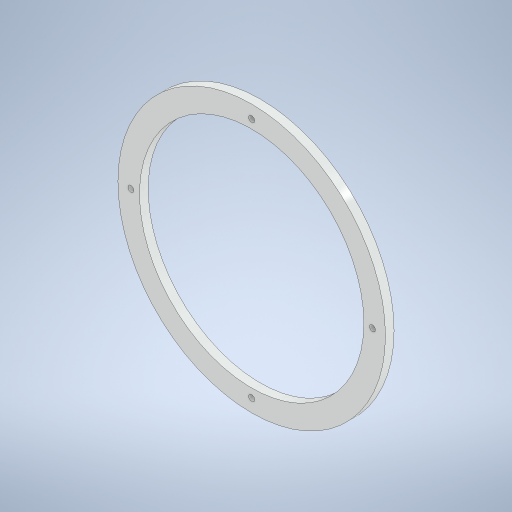
# Autodesk Inventor part: 아크릴 고정판
Saved by Autodesk Inventor 2023.1 (Build 271208000, 208)
## iProperties
Created: 2022-08-14
Part Number: 아크릴 고정판
Material: 일반
Document SubType Name: Modeling
Designer: fly01
Density: 1 g/cm^3
Appearance: 기본값
Author: fly01
Autodesk Inventor part; units mm, degrees
ref_plane "YZ Plane" through (0, 0, 0) normal (1, 0, 0) x (0, 1, 0)
ref_plane "XZ Plane" through (0, 0, 0) normal (0, 1, 0) x (-1, 0, 0)
ref_plane "XY Plane" through (0, 0, 0) normal (0, 0, 1) x (1, 0, 0)
sketch "스케치1" plane through (0, 0, 0) normal (0, 0, 1) x (1, 0, 0)
  circle A0 centre (0, 0) radius 77.5
  circle A1 centre (0, 0) radius 65
  dimension "d0" = 155
  dimension "d1" = 130
  constraints: 2 centre point, 2 coincident
  measures "d0" diameter of A0
  measures "d1" diameter of A1
extrude "돌출1" add sketch "스케치1" along normal blind 5
sketch "스케치2" plane through (0, 0, 5) normal (0, 0, 1) x (1, 0, 0)
  circle A0 centre (0, 70) radius 1.75
  circle A1 centre (-70, 0) radius 1.75
  circle A2 centre (0, -70) radius 1.75
  circle A3 centre (70, 0) radius 1.75
  point P0 (0, 0)
  dimension "d4" = 3.5
  dimension "d5" = 70
  dimension "d8" = 360
  constraints: 4 centre point, 9 other
  measures "d4" diameter of A0
  measures "d5" distance of point (0, 0) A0.centre
extrude "돌출2" cut sketch "스케치2" against normal blind 5
